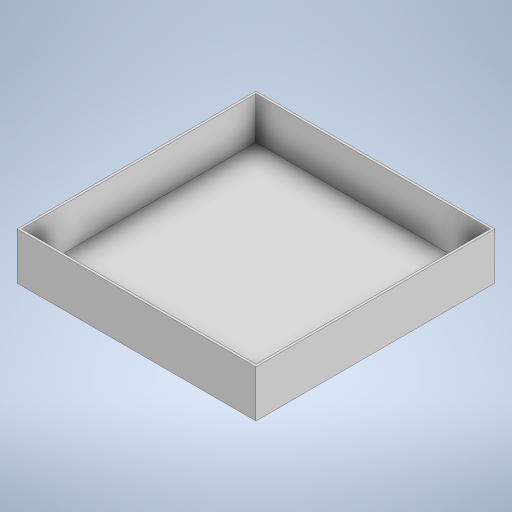
# Autodesk Inventor part: box
Saved by Autodesk Inventor 2024 (Build 280153000, 153)
## iProperties
Created: 2023-11-14
Part Number: box
Material: Všeobecné
Document SubType Name: Modeling
Designer: Simak
Density: 1 g/cm^3
Appearance: Výchozí
Author: Simak
Autodesk Inventor part; units mm, degrees
ref_plane "YZ Plane" through (0, 0, 0) normal (1, 0, 0) x (0, 1, 0)
ref_plane "XZ Plane" through (0, 0, 0) normal (0, 1, 0) x (-1, 0, 0)
ref_plane "XY Plane" through (0, 0, 0) normal (0, 0, 1) x (1, 0, 0)
sketch "Náčrt1" plane through (0, 0, 0) normal (0, 1, 0) x (-1, 0, 0)
  line L0 (102, 0) -> (0, 0)
  line L1 (0, 0) -> (0, -102)
  line L2 (0, -102) -> (102, -102)
  line L3 (102, -102) -> (102, 0)
  dimension "d0" = 102
  constraints: 8 end point, 2 parallel, 2 perpendicular, 1 coincident, 1 horizontal
  measures "d0" distance of L2.end L0.start
extrude "Vysunutí1" add sketch "Náčrt1" along normal blind 20
sketch "Náčrt2" plane through (0, 20, 0) normal (0, 1, 0) x (1, 0, 0)
  line L0 (0, 0) -> (0, 102) projected
  line L1 (0, 102) -> (-102, 102) projected
  line L2 (-102, 102) -> (-102, 0) projected
  line L3 (-102, 0) -> (0, 0) projected
  line L4 (-101, 1) -> (-101, 101)
  line L5 (-101, 101) -> (-1, 101)
  line L6 (-1, 101) -> (-1, 1)
  line L7 (-1, 1) -> (-101, 1)
  dimension "d3" = 1
  constraints: 8 end point, 3 other
  measures "d3" distance between parallel lines of L2 L4
extrude "Vysunutí2" cut sketch "Náčrt2" against normal blind 18 contours L4 L5 L6 L7
